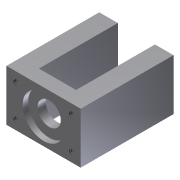
# Autodesk Inventor part: mount pillow block inner
Saved by Autodesk Inventor 2012 (Build 160160000, 160)
## iProperties
Created: 2012-04-26
Part Number: mount pillow block inner
Material: Default
Document SubType Name: Modeling
Designer: Antonella Wilby
Density: 1 g/cm^3
Author: Antonella Wilby
Autodesk Inventor part; units mm, degrees
ref_plane "YZ Plane" through (0, 0, 0) normal (1, 0, 0) x (0, 1, 0)
ref_plane "XZ Plane" through (0, 0, 0) normal (0, 1, 0) x (-1, 0, 0)
ref_plane "XY Plane" through (0, 0, 0) normal (0, 0, 1) x (1, 0, 0)
sketch "Sketch1" plane through (0, 0, 0) normal (0, 0, 1) x (1, 0, 0)
  line L0 (-35.56, 0) -> (35.56, 0) projected
  line L1 (0, -24.4475) -> (0, 24.4475) projected
  circle A0 centre (0, 0) radius 14.2875 construction
  line L2 (-25.4, 17.4625) -> (25.4, 17.4625)
  line L3 (25.4, 17.4625) -> (25.4, -17.4625)
  line L4 (25.4, -17.4625) -> (-25.4, -17.4625)
  line L5 (-25.4, -17.4625) -> (-25.4, 17.4625)
  circle A1 centre (0, 0) radius 7.9375
  point P0 (0, 17.4625)
  point P1 (25.4, 0)
  dimension "d1" = 28.575
  dimension "d2" = 34.925
  dimension "d3" = 50.8
  dimension "d4" = 15.875
  constraints: 8 end point, 2 centre point, 2 coincident, 2 midpoint, 2 parallel, 1 horizontal, 1 horizontal alignment, 1 perpendicular, 1 vertical alignment
  measures "d1" diameter of A0
  measures "d2" distance of L2.end L3.end
  measures "d3" distance of L3.end L4.end
  measures "d4" diameter of A1
extrude "Extrusion1" add sketch "Sketch1" against normal blind 63.5 contours L5 L2 L1 A1 L0 | L0 A1 L1 L4 L5 | L1 L2 L3 L0 A1 | A1 L0 L3 L4 L1
sketch "Sketch2" plane through (0, 0, -63.5) normal (0, 0, -1) x (-1, 0, 0)
  circle A0 centre (0, 0) radius 7.9375 projected
  line L0 (-25.4, 17.4625) -> (25.4, 17.4625) projected
  line L1 (25.4, -17.4625) -> (-25.4, -17.4625) projected
  line L2 (-12.7, 17.4625) -> (12.7, 17.4625)
  line L3 (12.7, 17.4625) -> (12.7, -17.4625)
  line L4 (12.7, -17.4625) -> (-12.7, -17.4625)
  line L5 (-12.7, -17.4625) -> (-12.7, 17.4625)
  point P0 (0, 17.4625)
  point P1 (0, 17.4625)
  dimension "d7" = 25.4
  constraints: 8 end point, 2 midpoint, 2 parallel, 2 point on line, 2 vertical alignment, 1 horizontal, 1 perpendicular
  measures "d7" distance between parallel lines of L3 L5
extrude "Extrusion2" cut sketch "Sketch2" against normal blind 53.975
sketch "Sketch3" plane through (0, 0, 0) normal (0, 0, 1) x (1, 0, 0)
  circle A0 centre (0, 0) radius 7.9375 projected
  circle A1 centre (0, 0) radius 14.3256
  dimension "d10" = 28.6512
  constraints: 1 centre point, 1 coincident
  measures "d10" diameter of A1
extrude "Extrusion3" cut sketch "Sketch3" against normal blind 3.81
sketch "Sketch5" plane through (0, 0, 0) normal (0, 0, 1) x (1, 0, 0)
  line L0 (-25.4, 17.4625) -> (25.4, 17.4625) projected
  line L1 (-25.4, -17.4625) -> (-25.4, 17.4625) projected
  line L2 (-35.56, 0) -> (35.56, 0) projected
  line L3 (0, -24.4475) -> (0, 24.4475) projected
  point P0 (-19.05, 11.1125)
  point P1 (19.05, 11.1125)
  point P2 (-19.05, -11.1125)
  point P3 (19.05, -11.1125)
  dimension "d13" = 6.35
  dimension "d14" = 6.35
  constraints: 3 symmetric about line
  measures "d13" distance from line of L0 point (-19.05, 11.113)
  measures "d14" distance from line of L1 point (-19.05, 11.113)
hole "Hole1" at (-19.05, 11.1125, 0) at (19.05, 11.1125, 0) at (-19.05, -11.1125, 0) at (19.05, -11.1125, 0) direction (0, 0, -1) diameter 3.683 depth 19.05 tip angle 118 thread size "10-24 UNC" class "2B" standard "ANSI Unified Screw Threads"
sketch "Sketch6" plane through (0, 0, -63.5) normal (0, 0, -1) x (-1, 0, 0)
  line L0 (12.7, 17.4625) -> (25.4, 17.4625) projected
  line L1 (35.56, 0) -> (-35.56, 0) projected
  line L2 (0, -24.4475) -> (0, 24.4475) projected
  point P0 (0, 0)
  point P1 (19.05, 11.1125)
  point P2 (19.05, 17.4625)
  point P3 (19.05, -11.1125)
  dimension "d22" = 6.35
  constraints: 1 midpoint, 1 symmetric about line, 1 vertical alignment
  measures "d22" distance from line of L0 point (19.05, 11.113)
hole "Hole2" at (-19.05, 11.1125, -63.5) at (-19.05, -11.1125, -63.5) direction (0, 0, 1) diameter 3.683 depth 19.05 tip angle 118 thread size "10-24 UNC" class "2B" standard "ANSI Unified Screw Threads"
mirror "Mirror1" about plane through (0, 0, 0) normal (1, 0, 0) of "Hole2"
body "Solid1"
